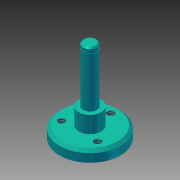
# Autodesk Inventor part: 13_0204_017
Saved by Autodesk Inventor 2012 SP1 (Build 160190100, 190)
## iProperties
Created: 2013-03-21
Part Number: 13_0204_017
Material: Default
Document SubType Name: Modeling
Designer: vogel
Density: 1 g/cm^3
Author: vogel
Autodesk Inventor part; units mm, degrees
ref_plane "YZ Plane" through (0, 0, 0) normal (1, 0, 0) x (0, 1, 0)
ref_plane "XZ Plane" through (0, 0, 0) normal (0, 1, 0) x (-1, 0, 0)
ref_plane "XY Plane" through (0, 0, 0) normal (0, 0, 1) x (1, 0, 0)
sketch "Skizze1" plane through (0, 0, 0) normal (0, 0, 1) x (1, 0, 0)
  circle A0 centre (0, 0) radius 11
  dimension "d0" = 22
  constraints: 1 centre point, 1 coincident
  measures "d0" diameter of A0
extrude "Extrusion1" add sketch "Skizze1" along normal blind 4
sketch "Skizze2" plane through (0, 0, 4) normal (0, 0, 1) x (1, 0, 0)
  circle A0 centre (0, 0) radius 11 projected
  circle A1 centre (0, 0) radius 4
  dimension "d3" = 8
  constraints: 1 centre point, 1 coincident
  measures "d3" diameter of A1
extrude "Extrusion2" add sketch "Skizze2" along normal blind 6 contours A1
sketch "Skizze3" plane through (0, 0, 10) normal (0, 0, 1) x (1, 0, 0)
  circle A0 centre (0, 0) radius 4 projected
  circle A1 centre (0, 0) radius 2.5
  dimension "d6" = 5
  constraints: 1 centre point, 1 coincident
  measures "d6" diameter of A1
extrude "Extrusion3" add sketch "Skizze3" along normal blind 20 contours A1
sketch "Skizze4" plane through (0, 0, 0) normal (0, 0, -1) x (-1, 0, 0)
  circle A0 centre (0, 0) radius 11 projected
  line L0 (17.5, 0) -> (-17.5, 0) projected
  line L1 (0, -17.5) -> (0, 17.5) projected
  circle A1 centre (0, 0) radius 7.5
  line L2 (6.4952, -3.75) -> (0, 0)
  line L3 (0, 0) -> (-6.4952, -3.75)
  point P0 (0, 7.5)
  dimension "d9" = 15
  dimension "d10" = 120
  dimension "d11" = 120
  constraints: 4 end point, 3 point on circle, 1 centre point, 1 coincident, 1 point on line
  measures "d9" diameter of A1
  measures "d10" angle of L2 L1
  measures "d11" angle of L3 L1
hole "Bohrung1" at (0, 7.5, 0) at (-6.4952, -3.75, 0) at (6.4952, -3.75, 0) direction (0, 0, 1) diameter 2.459 end through all thread size "M3x0.5" class "6H" standard "ISO Metric profile"
chamfer "Fase1" distance 0.5 angle 45 1 edges at (-2.5, 0, 30)
sketch "Skizze5" plane through (0, 0, 0) normal (1, 0, 0) x (0, 1, 0)
  line L0 (-2.5, 10) -> (2.5, 10) projected
  line L1 (2.5, 29.5) -> (-2.5, 29.5) projected
  line L2 (2.5, 10) -> (2.5, 29.5) projected
  line L3 (0, -4.3) -> (0, 25.8) projected
  line L4 (2.5, 28.7) -> (2.4, 28.7)
  line L5 (2.4, 28.7) -> (2.4, 28)
  line L6 (2.4, 28) -> (2.5, 28)
  line L7 (2.5, 28) -> (2.5, 28.7)
  point P0 (0, 0)
  dimension "d31" = 18
  dimension "d32" = 0.7
  dimension "d33" = 4.8
  constraints: 8 end point, 2 parallel, 1 horizontal, 1 perpendicular, 1 point on line
  measures "d31" distance between parallel lines of L6 L0
  measures "d32" distance between parallel lines of L4 L6
  measures "d33" diameter of L5 L3
revolve "Umdrehung1" cut sketch "Skizze5" angle 360 about axis through (0, 0, -10) along (0, 0, 1)
chamfer "Fase3" distance 1 angle 45 1 edges at (-11, 0, 4)
